Autodesk Inventor part; units mm, degrees
(part 6 of 6)
  line L2705 (-92.0833, 59.5046) -> (-92.092, 59.5384) projected
  line L2706 (-92.092, 59.5384) -> (-92.1001, 59.5723) projected
  line L2707 (-92.1001, 59.5723) -> (-92.1077, 59.6064) projected
  line L2708 (-92.1077, 59.6064) -> (-92.1147, 59.6406) projected
  line L2709 (-92.1147, 59.6406) -> (-92.121, 59.6749) projected
  line L2710 (-92.121, 59.6749) -> (-92.1268, 59.7093) projected
  line L2711 (-92.1268, 59.7093) -> (-92.1319, 59.7439) projected
  line L2712 (-92.1319, 59.7439) -> (-92.1365, 59.7785) projected
  line L2713 (-92.1365, 59.7785) -> (-92.1404, 59.8131) projected
  line L2714 (-92.1404, 59.8131) -> (-92.1438, 59.8479) projected
  line L2715 (-92.1438, 59.8479) -> (-92.1465, 59.8827) projected
  line L2716 (-92.1465, 59.8827) -> (-92.1487, 59.9175) projected
  line L2717 (-92.1487, 59.9175) -> (-92.1502, 59.9524) projected
  line L2718 (-92.1502, 59.9524) -> (-92.1511, 59.9873) projected
  line L2719 (-92.1511, 59.9873) -> (-92.1514, 60.0222) projected
  line L2720 (-92.1514, 60.0222) -> (-92.1511, 60.0571) projected
  line L2721 (-92.1511, 60.0571) -> (-92.1502, 60.092) projected
  line L2722 (-92.1502, 60.092) -> (-92.1487, 60.1269) projected
  line L2723 (-92.1487, 60.1269) -> (-92.1465, 60.1617) projected
  line L2724 (-92.1465, 60.1617) -> (-92.1438, 60.1965) projected
  line L2725 (-92.1438, 60.1965) -> (-92.1404, 60.2313) projected
  line L2726 (-92.1404, 60.2313) -> (-92.1365, 60.2659) projected
  line L2727 (-92.1365, 60.2659) -> (-92.1319, 60.3005) projected
  line L2728 (-92.1319, 60.3005) -> (-92.1268, 60.3351) projected
  line L2729 (-92.1268, 60.3351) -> (-92.121, 60.3695) projected
  line L2730 (-92.121, 60.3695) -> (-92.1147, 60.4038) projected
  line L2731 (-92.1147, 60.4038) -> (-92.1077, 60.438) projected
  line L2732 (-92.1077, 60.438) -> (-92.1001, 60.4721) projected
  line L2733 (-92.1001, 60.4721) -> (-92.092, 60.506) projected
  line L2734 (-92.092, 60.506) -> (-92.0833, 60.5398) projected
  line L2735 (-92.0833, 60.5398) -> (-92.0739, 60.5735) projected
  line L2736 (-92.0739, 60.5735) -> (-92.064, 60.6069) projected
  line L2737 (-92.064, 60.6069) -> (-92.0535, 60.6402) projected
  line L2738 (-92.0535, 60.6402) -> (-92.0424, 60.6733) projected
  line L2739 (-92.0424, 60.6733) -> (-92.0308, 60.7062) projected
  line L2740 (-92.0308, 60.7062) -> (-92.0186, 60.7389) projected
  line L2741 (-92.0186, 60.7389) -> (-92.0058, 60.7714) projected
  line L2742 (-92.0058, 60.7714) -> (-91.9924, 60.8037) projected
  line L2743 (-91.9924, 60.8037) -> (-91.9785, 60.8357) projected
  line L2744 (-91.9785, 60.8357) -> (-91.964, 60.8674) projected
  line L2745 (-91.964, 60.8674) -> (-91.949, 60.8989) projected
  line L2746 (-91.949, 60.8989) -> (-91.9334, 60.9302) projected
  line L2747 (-91.9334, 60.9302) -> (-91.9173, 60.9611) projected
  line L2748 (-91.9173, 60.9611) -> (-91.9006, 60.9918) projected
  line L2749 (-91.9006, 60.9918) -> (-91.8835, 61.0222) projected
  line L2750 (-91.8835, 61.0222) -> (-91.8657, 61.0523) projected
  line L2751 (-91.8657, 61.0523) -> (-91.8475, 61.082) projected
  line L2752 (-91.8475, 61.082) -> (-91.8287, 61.1115) projected
  line L2753 (-91.8287, 61.1115) -> (-91.8095, 61.1406) projected
  line L2754 (-91.8095, 61.1406) -> (-91.7897, 61.1694) projected
  line L2755 (-91.7897, 61.1694) -> (-91.7694, 61.1978) projected
  line L2756 (-91.7694, 61.1978) -> (-91.7487, 61.2258) projected
  line L2757 (-91.7487, 61.2258) -> (-91.7274, 61.2535) projected
  line L2758 (-91.7274, 61.2535) -> (-91.7057, 61.2808) projected
  line L2759 (-91.7057, 61.2808) -> (-91.6835, 61.3078) projected
  line L2760 (-91.6835, 61.3078) -> (-91.6608, 61.3343) projected
  line L2761 (-91.6608, 61.3343) -> (-91.6377, 61.3605) projected
  line L2762 (-91.6377, 61.3605) -> (-91.6141, 61.3862) projected
  line L2763 (-91.6141, 61.3862) -> (-91.5901, 61.4115) projected
  line L2764 (-91.5901, 61.4115) -> (-91.5656, 61.4364) projected
  line L2765 (-91.5656, 61.4364) -> (-91.5407, 61.4609) projected
  line L2766 (-91.5407, 61.4609) -> (-91.5154, 61.4849) projected
  line L2767 (-91.5154, 61.4849) -> (-91.4897, 61.5085) projected
  line L2768 (-91.4897, 61.5085) -> (-91.4635, 61.5316) projected
  line L2769 (-91.4635, 61.5316) -> (-91.437, 61.5543) projected
  line L2770 (-91.437, 61.5543) -> (-91.41, 61.5765) projected
  line L2771 (-91.41, 61.5765) -> (-91.3827, 61.5982) projected
  line L2772 (-91.3827, 61.5982) -> (-91.355, 61.6195) projected
  line L2773 (-91.355, 61.6195) -> (-91.327, 61.6402) projected
  line L2774 (-91.327, 61.6402) -> (-91.2986, 61.6605) projected
  line L2775 (-91.2986, 61.6605) -> (-91.2698, 61.6803) projected
  line L2776 (-91.2698, 61.6803) -> (-91.2407, 61.6995) projected
  line L2777 (-91.2407, 61.6995) -> (-91.2112, 61.7183) projected
  line L2778 (-91.2112, 61.7183) -> (-91.1815, 61.7365) projected
  line L2779 (-91.1815, 61.7365) -> (-91.1514, 61.7543) projected
  line L2780 (-91.1514, 61.7543) -> (-91.121, 61.7714) projected
  line L2781 (-91.121, 61.7714) -> (-91.0904, 61.7881) projected
  line L2782 (-91.0904, 61.7881) -> (-91.0594, 61.8042) projected
  line L2783 (-91.0594, 61.8042) -> (-91.0282, 61.8198) projected
  line L2784 (-91.0282, 61.8198) -> (-90.9966, 61.8348) projected
  line L2785 (-90.9966, 61.8348) -> (-90.9649, 61.8493) projected
  line L2786 (-90.9649, 61.8493) -> (-90.9329, 61.8632) projected
  line L2787 (-90.9329, 61.8632) -> (-90.9006, 61.8766) projected
  line L2788 (-90.9006, 61.8766) -> (-90.8681, 61.8894) projected
  line L2789 (-90.8681, 61.8894) -> (-90.8354, 61.9016) projected
  line L2790 (-90.8354, 61.9016) -> (-90.8025, 61.9132) projected
  line L2791 (-90.8025, 61.9132) -> (-90.7694, 61.9243) projected
  line L2792 (-90.7694, 61.9243) -> (-90.7362, 61.9348) projected
  line L2793 (-90.7362, 61.9348) -> (-90.7027, 61.9447) projected
  line L2794 (-90.7027, 61.9447) -> (-90.669, 61.9541) projected
  line L2795 (-90.669, 61.9541) -> (-90.6353, 61.9628) projected
  line L2796 (-90.6353, 61.9628) -> (-90.6013, 61.9709) projected
  line L2797 (-90.6013, 61.9709) -> (-90.5672, 61.9785) projected
  line L2798 (-90.5672, 61.9785) -> (-90.533, 61.9855) projected
  line L2799 (-90.533, 61.9855) -> (-90.4987, 61.9918) projected
  line L2800 (-90.4987, 61.9918) -> (-90.4643, 61.9976) projected
  line L2801 (-90.4643, 61.9976) -> (-90.4298, 62.0027) projected
  line L2802 (-90.4298, 62.0027) -> (-90.3951, 62.0073) projected
  line L2803 (-90.3951, 62.0073) -> (-90.3605, 62.0112) projected
  line L2804 (-90.3605, 62.0112) -> (-90.3257, 62.0146) projected
  line L2805 (-90.3257, 62.0146) -> (-90.2909, 62.0173) projected
  line L2806 (-90.2909, 62.0173) -> (-90.2561, 62.0195) projected
  line L2807 (-90.2561, 62.0195) -> (-90.2212, 62.021) projected
  line L2808 (-90.2212, 62.021) -> (-90.1863, 62.0219) projected
  line L2809 (-90.1863, 62.0219) -> (-90.1514, 62.0222) projected
  line L2810 (-90.1514, 62.0222) -> (-90.1165, 62.0219) projected
  line L2811 (-90.1165, 62.0219) -> (-90.0816, 62.021) projected
  line L2812 (-90.0816, 62.021) -> (-90.0467, 62.0195) projected
  line L2813 (-90.0467, 62.0195) -> (-90.0119, 62.0173) projected
  line L2814 (-90.0119, 62.0173) -> (-89.9771, 62.0146) projected
  line L2815 (-89.9771, 62.0146) -> (-89.9424, 62.0112) projected
  line L2816 (-89.9424, 62.0112) -> (-89.9077, 62.0073) projected
  line L2817 (-89.9077, 62.0073) -> (-89.8731, 62.0027) projected
  line L2818 (-89.8731, 62.0027) -> (-89.8385, 61.9976) projected
  line L2819 (-89.8385, 61.9976) -> (-89.8041, 61.9918) projected
  line L2820 (-89.8041, 61.9918) -> (-89.7698, 61.9855) projected
  line L2821 (-89.7698, 61.9855) -> (-89.7356, 61.9785) projected
  line L2822 (-89.7356, 61.9785) -> (-89.7015, 61.9709) projected
  line L2823 (-89.7015, 61.9709) -> (-89.6676, 61.9628) projected
  line L2824 (-89.6676, 61.9628) -> (-89.6338, 61.9541) projected
  line L2825 (-89.6338, 61.9541) -> (-89.6001, 61.9447) projected
  line L2826 (-89.6001, 61.9447) -> (-89.5667, 61.9348) projected
  line L2827 (-89.5667, 61.9348) -> (-89.5334, 61.9243) projected
  line L2828 (-89.5334, 61.9243) -> (-89.5003, 61.9132) projected
  line L2829 (-89.5003, 61.9132) -> (-89.4674, 61.9016) projected
  line L2830 (-89.4674, 61.9016) -> (-89.4347, 61.8894) projected
  line L2831 (-89.4347, 61.8894) -> (-89.4022, 61.8766) projected
  line L2832 (-89.4022, 61.8766) -> (-89.3699, 61.8632) projected
  line L2833 (-89.3699, 61.8632) -> (-89.3379, 61.8493) projected
  line L2834 (-89.3379, 61.8493) -> (-89.3062, 61.8348) projected
  line L2835 (-89.3062, 61.8348) -> (-89.2747, 61.8198) projected
  line L2836 (-89.2747, 61.8198) -> (-89.2434, 61.8042) projected
  line L2837 (-89.2434, 61.8042) -> (-89.2125, 61.7881) projected
  line L2838 (-89.2125, 61.7881) -> (-89.1818, 61.7714) projected
  line L2839 (-89.1818, 61.7714) -> (-89.1514, 61.7543) projected
  line L2840 (-89.1514, 61.7543) -> (-89.1213, 61.7365) projected
  line L2841 (-89.1213, 61.7365) -> (-89.0916, 61.7183) projected
  line L2842 (-89.0916, 61.7183) -> (-89.0621, 61.6995) projected
  line L2843 (-89.0621, 61.6995) -> (-89.033, 61.6803) projected
  line L2844 (-89.033, 61.6803) -> (-89.0043, 61.6605) projected
  line L2845 (-89.0043, 61.6605) -> (-88.9758, 61.6402) projected
  line L2846 (-88.9758, 61.6402) -> (-88.9478, 61.6195) projected
  line L2847 (-88.9478, 61.6195) -> (-88.9201, 61.5982) projected
  line L2848 (-88.9201, 61.5982) -> (-88.8928, 61.5765) projected
  line L2849 (-88.8928, 61.5765) -> (-88.8658, 61.5543) projected
  line L2850 (-88.8658, 61.5543) -> (-88.8393, 61.5316) projected
  line L2851 (-88.8393, 61.5316) -> (-88.8132, 61.5085) projected
  line L2852 (-88.8132, 61.5085) -> (-88.7874, 61.4849) projected
  line L2853 (-88.7874, 61.4849) -> (-88.7621, 61.4609) projected
  line L2854 (-88.7621, 61.4609) -> (-88.7372, 61.4364) projected
  line L2855 (-88.7372, 61.4364) -> (-88.7127, 61.4115) projected
  line L2856 (-88.7127, 61.4115) -> (-88.6887, 61.3862) projected
  line L2857 (-88.6887, 61.3862) -> (-88.6651, 61.3605) projected
  line L2858 (-88.6651, 61.3605) -> (-88.642, 61.3343) projected
  line L2859 (-88.642, 61.3343) -> (-88.6193, 61.3078) projected
  line L2860 (-88.6193, 61.3078) -> (-88.5971, 61.2808) projected
  line L2861 (-88.5971, 61.2808) -> (-88.5754, 61.2535) projected
  line L2862 (-88.5754, 61.2535) -> (-88.5541, 61.2258) projected
  line L2863 (-88.5541, 61.2258) -> (-88.5334, 61.1978) projected
  line L2864 (-88.5334, 61.1978) -> (-88.5131, 61.1694) projected
  line L2865 (-88.5131, 61.1694) -> (-88.4933, 61.1406) projected
  line L2866 (-88.4933, 61.1406) -> (-88.4741, 61.1115) projected
  line L2867 (-88.4741, 61.1115) -> (-88.4553, 61.082) projected
  line L2868 (-88.4553, 61.082) -> (-88.4371, 61.0523) projected
  line L2869 (-88.4371, 61.0523) -> (-88.4194, 61.0222) projected
  line L2870 (-88.4194, 61.0222) -> (-88.4022, 60.9918) projected
  line L2871 (-88.4022, 60.9918) -> (-88.3855, 60.9611) projected
  line L2872 (-88.3855, 60.9611) -> (-88.3694, 60.9302) projected
  line L2873 (-88.3694, 60.9302) -> (-88.3538, 60.8989) projected
  line L2874 (-88.3538, 60.8989) -> (-88.3388, 60.8674) projected
  line L2875 (-88.3388, 60.8674) -> (-88.3243, 60.8357) projected
  line L2876 (-88.3243, 60.8357) -> (-88.3104, 60.8037) projected
  line L2877 (-88.3104, 60.8037) -> (-88.297, 60.7714) projected
  line L2878 (-88.297, 60.7714) -> (-88.2843, 60.7389) projected
  line L2879 (-88.2843, 60.7389) -> (-88.272, 60.7062) projected
  line L2880 (-88.272, 60.7062) -> (-88.2604, 60.6733) projected
  line L2881 (-88.2604, 60.6733) -> (-88.2493, 60.6402) projected
  line L2882 (-88.2493, 60.6402) -> (-88.2388, 60.6069) projected
  line L2883 (-88.2388, 60.6069) -> (-88.2289, 60.5735) projected
  line L2884 (-88.2289, 60.5735) -> (-88.2196, 60.5398) projected
  line L2885 (-88.2196, 60.5398) -> (-88.2108, 60.506) projected
  line L2886 (-88.2108, 60.506) -> (-88.2027, 60.4721) projected
  line L2887 (-88.2027, 60.4721) -> (-88.1951, 60.438) projected
  line L2888 (-88.1951, 60.438) -> (-88.1882, 60.4038) projected
  line L2889 (-88.1882, 60.4038) -> (-88.1818, 60.3695) projected
  line L2890 (-88.1818, 60.3695) -> (-88.176, 60.3351) projected
  line L2891 (-88.176, 60.3351) -> (-88.1709, 60.3005) projected
  line L2892 (-88.1709, 60.3005) -> (-88.1663, 60.2659) projected
  line L2893 (-88.1663, 60.2659) -> (-88.1624, 60.2313) projected
  line L2894 (-88.1624, 60.2313) -> (-88.159, 60.1965) projected
  line L2895 (-88.159, 60.1965) -> (-88.1563, 60.1617) projected
  point P0 (0, 0)
  point P1 (-90.1577, 58.0222)
  point P2 (-90.1577, -57.9779)
  point P3 (-88.152, -60.0222)
  point P4 (87.849, -60.0222)
  point P5 (90.1577, -58.0019)
  point P6 (90.1577, 58.0462)
  dimension "d14" = 5
  dimension "d15" = 5
  constraints: 12 end point, 2 midpoint, 2 parallel, 1 horizontal, 1 perpendicular
  measures "d14" distance between parallel lines of L2 L6
  measures "d15" distance between parallel lines of L9 L3
extrude "Extrusão3" cut sketch "Esboço4" against normal through all contours L732 L731 L1090 L1089 L1088 L1087 L1086 L1085 L1084 L1083 L1082 L1081 L1080 L1079 L1078 L1077 L1076 L1075 L1074 L1073 L1072 L1071 L1070 L1069 L1068 L1067 L1066 L1065 L1064 L1063 L1062 L1061 L1060 L1059 L1058 L1057 L1056 L1055 L1054 L1053 L1052 L1051 L1050 L1049 L1048 L1047 L1046 L1045 L1044 L1043 L1042 L1041 L1040 L1039 L1038 L1037 L1036 L1035 L1034 L1033 L1032 L1031 L1030 L1029 L1028 L1027 L1026 L1025 L1024 L1023 L1022 L1021 L1020 L1019 L1018 L1017 L1016 L1015 L1014 L1013 L1012 L1011 L1010 L1009 L1008 L1007 L1006 L1005 L1004 L1003 L1002 L1001 L1000 L3 L1185 L1184 L1183 L1182 L1181 L1180 L1179 L1178 L1177 L1176 L1175 L1174 L1173 L1172 L1171 L1170 L1169 L1168 L1167 L1166 L1165 L1164 L1163 L1162 L1161 L1160 L1159 L1158 L1157 L1156 L1155 L1154 L1153 L1152 L1151 L1150 L1149 L1148 L1147 L1146 L1145 L1144 L1143 L1142 L1141 L1140 L1139 L1138 L1137 L1136 L1135 L1134 L1133 L1132 L1131 L1130 L1129 L1128 L1127 L1126 L1125 L1124 L1123 L1122 L1121 L1120 L1119 L1118 L1117 L1116 L1115 L1114 L1113 L1112 L1111 L1110 L1109 L1108 L1107 L1106 L1105 L1104 L1103 L1102 L1101 L1100 L1099 L1098 L1097 L1096 L1095 L2 L190 L189 L188 L187 L186 L185 L184 L183 L182 L181 L180 L179 L178 L177 L176 L175 L174 L173 L172 L171 L170 L169 L168 L167 L166 L165 L164 L163 L162 L161 L160 L159 L158 L157 L156 L155 L154 L153 L152 L151 L150 L149 L148 L147 L146 L145 L144 L143 L142 L141 L140 L139 L138 L137 L136 L135 L134 L133 L132 L131 L130 L129 L128 L127 L126 L125 L124 L123 L122 L121 L120 L119 L118 L117 L116 L115 L114 L113 L112 L111 L110 L109 L108 L107 L106 L105 L104 L103 L102 L101 L100 L99 L98 L97 L96 L95 L94 L93 L92 L1 L649 L648 L647 L646 L645 L644 L643 L642 L641 L640 L639 L638 L637 L636 L635 L634 L633 L632 L631 L630 L629 L628 L627 L626 L625 L624 L623 L622 L621 L620 L619 L618 L617 L616 L615 L614 L613 L612 L611 L610 L609 L608 L607 L606 L605 L604 L603 L602 L601 L600 L599 L598 L597 L596 L595 L594 L593 L592 L591 L590 L589 L588 L587 L586 L585 L584 L583 L582 L581 L580 L579 L578 L577 L576 L575 L574 L573 L572 L571 L570 L569 L568 L567 L566 L565 L564 L563 L562 L561 L560 L559 L558 L557 L556 L555 L554 L553 L552 L551 L550 L549 L0
sketch "Esboço5" plane through (0, 0, 8) normal (0, 0, 1) x (1, 0, 0)
  line L0 (87.849, -60.0222) -> (-88.152, -60.0222) projected
  line L1 (91.8482, -60.0127) -> (91.8473, -60.0476) projected
  point P0 (0, 0)
sketch "Esboço6" plane through (0, 0, 8) normal (0, 0, 1) x (1, 0, 0)
  line L0 (87.849, -60.0222) -> (-88.152, -60.0222) projected
  circle A0 centre (-90.1448, -59.9677) radius 2
  circle A1 centre (-90.1448, -59.9677) radius 4
  line L1 (-90.1577, -57.9779) -> (-90.1577, 58.0222) projected
  line L2 (-90.1577, 0.0222) -> (90.1577, 0.0222)
  line L3 (90.1577, 58.0462) -> (90.1577, -58.0019) projected
  line L4 (-88.1514, 60.0222) -> (87.8485, 60.0222) projected
  line L5 (-0.1515, 60.0222) -> (-0.1515, -60.0222)
  circle A2 centre (89.8419, -59.9677) radius 2
  circle A3 centre (89.8419, -59.9677) radius 4
  line L6 (87.849, 60.0665) -> (-88.152, 60.0665)
  circle A4 centre (-90.1448, 60.012) radius 2
  circle A5 centre (-90.1448, 60.012) radius 4
  circle A6 centre (89.8419, 60.012) radius 2
  circle A7 centre (89.8419, 60.012) radius 4
  point P0 (0, 0)
  point P1 (89.8548, -57.9779)
  point P2 (-0.1515, 60.0665)
  point P3 (89.8548, 58.0222)
  point P4 (90.1577, -55.9802)
  point P5 (85.8422, -60.0222)
  point P6 (87.8426, -60.0222)
  point P7 (90.1577, -57.9928)
  point P8 (-90.1577, -55.9677)
  point P9 (-90.1577, -57.9677)
  point P10 (-88.1456, -60.0222)
  point P11 (-86.1452, -60.0222)
  point P12 (-86.1448, 60.0222)
  point P13 (-88.1448, 60.0222)
  point P14 (-90.1577, 58.0121)
  point P15 (-90.1577, 56.012)
  point P16 (85.8419, 60.0222)
  point P17 (90.1577, 56.0245)
  point P18 (90.1577, 58.0371)
  point P19 (87.8419, 60.0222)
  dimension "d18" = 8
  dimension "d19" = 4
  constraints: 11 symmetric about line, 8 centre point, 6 end point, 4 coincident, 4 midpoint, 6 other
  measures "d18" diameter of A1
  measures "d19" diameter of A0
extrude "Extrusão4" add sketch "Esboço6" against normal up to surface (8 mm away) contours L0 A3 L3 A2 | L0 A0 L1 A1 | A7 L4 A6 L3 | L1 A4 L4 A5 picked at (86.5543, -59.5623) picked at (-86.845, -59.6704)
fillet "Arredondamento2" radius 2 8 edges at (90.1577, 56.0245, 4) (85.8419, 60.0222, 4) (90.1577, -55.9802, 4) (85.8422, -60.0222, 4) (-90.1577, -55.9677, 4) (-86.1452, -60.0222, 4) (-90.1577, 56.012, 4) (-86.1448, 60.0222, 4)
sketch "Esboço7" plane through (0, 0, 8) normal (0, 0, 1) x (1, 0, 0)
  circle A0 centre (-90.1448, 60.012) radius 2 projected
  arc A1 (87.8419, 60.0222) -> (90.1577, 58.0371) centre (89.8419, 60.012) ccw projected
  circle A2 centre (89.8419, 60.012) radius 2 projected
  circle A3 centre (89.8419, -59.9677) radius 2 projected
  circle A4 centre (-90.1448, -59.9677) radius 2 projected
  point P0 (0, 0)
extrude "Extrusão5" cut sketch "Esboço7" against normal through all
sketch "Esboço8" plane through (0, 0, 8) normal (0, 0, 1) x (1, 0, 0)
  arc A0 (88.1681, 61.1067) -> (91.5248, 58.9313) centre (89.8419, 60.012) ccw projected
  circle A1 centre (89.8419, 60.012) radius 2.5
  circle A2 centre (-90.1448, 60.012) radius 2.5
  arc A3 (-88.4741, -61.0671) -> (-91.8277, -58.887) centre (-90.1448, -59.9677) ccw projected
  circle A4 centre (-90.1448, -59.9677) radius 2.5
  arc A5 (91.5248, -58.887) -> (88.1681, -61.0624) centre (89.8419, -59.9677) ccw projected
  circle A6 centre (89.8419, -59.9677) radius 2.5
  point P0 (0, 0)
  dimension "d25" = 5
  dimension "d26" = 5
  dimension "d27" = 5
  dimension "d28" = 5
  constraints: 4 centre point, 4 coincident
  measures "d25" diameter of A6
  measures "d26" diameter of A1
  measures "d27" diameter of A2
  measures "d28" diameter of A4
extrude "Extrusão6" cut sketch "Esboço8" against normal blind 10
sketch "Esboço9" plane through (0, 0, 8) normal (0, 0, 1) x (1, 0, 0)
  circle A0 centre (-90.1448, 60.012) radius 2.5 projected
  circle A1 centre (-90.1448, 60.012) radius 1
  circle A2 centre (89.8419, 60.012) radius 2.5 projected
  circle A3 centre (89.8419, 60.012) radius 1
  circle A4 centre (89.8419, -59.9677) radius 2.5 projected
  circle A5 centre (89.8419, -59.9677) radius 1
  circle A6 centre (-90.1448, -59.9677) radius 2.5 projected
  circle A7 centre (-90.1448, -59.9677) radius 1
  point P0 (0, 0)
  dimension "d31" = 2
  dimension "d32" = 2
  dimension "d33" = 2
  dimension "d34" = 2
  constraints: 4 centre point, 4 coincident
  measures "d31" diameter of A7
  measures "d32" diameter of A5
  measures "d33" diameter of A3
  measures "d34" diameter of A1
extrude "Extrusão7" add sketch "Esboço9" against normal up to surface (8 mm away)
sketch "Esboço10" plane through (0, 0, 8) normal (0, 0, 1) x (1, 0, 0)
  circle A0 centre (-90.1448, 60.012) radius 1 projected
  circle A1 centre (89.8419, 60.012) radius 1 projected
  circle A2 centre (89.8419, -59.9677) radius 1 projected
  circle A3 centre (-90.1448, -59.9677) radius 1 projected
  point P0 (0, 0)
  constraints: 4 coincident
hole "Furo2" at (-90.1448, 60.012, 8) at (89.8419, 60.012, 8) at (89.8419, -59.9677, 8) at (-90.1448, -59.9677, 8) direction (0, 0, -1) diameter 3.242 end through all thread size "M4x0.7" class "6H" standard "ISO Metric profile"
